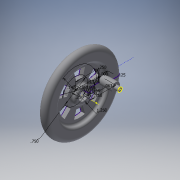
# Autodesk Inventor part: Caufield_Wheel
Saved by Autodesk Inventor 2016 (Build 200138000, 138)
## iProperties
Created: 2018-01-11
Part Number: Caufield_Wheel
Material: Generic
Document SubType Name: Modeling
Designer: The Panda
Density: 1 g/cm^3
Appearance: Default
Mass: 11.5444 g
Surface Area: 63.3015 cm^2
Volume: 11.5444 cm^3
Author: The Panda
Autodesk Inventor part; units mm, degrees
ref_plane "XZ Plane" through (0, 0, 0) normal (0, 1, 0) x (-1, 0, 0)
ref_plane "XY Plane" through (0, 0, 0) normal (0, 0, 1) x (1, 0, 0)
sketch "Wheel sketch" plane through (0, 0, 0) normal (0, 0, 1) x (1, 0, 0)
  line L0 (0, 0) -> (0, 6.4629) construction
  line L1 (3.556, 0) -> (3.556, 6.35)
  line L2 (25.4, 6.35) -> (25.4, 0) construction
  line L3 (25.4, 0) -> (3.556, 0)
  arc A0 (25.4, 0) -> (25.4, 6.35) centre (25.4, 3.175) ccw
  line L4 (0, 0) -> (43.9358, 0) construction
  line L5 (3.556, 6.35) -> (4.7625, 6.35)
  line L6 (6.35, 4.7625) -> (6.35, 4.7625)
  line L7 (7.9375, 3.175) -> (17.4625, 3.175)
  line L8 (25.4, 6.35) -> (20.6375, 6.35)
  line L9 (19.05, 4.7625) -> (19.05, 4.7625)
  arc A1 (6.35, 4.7625) -> (4.7625, 6.35) centre (4.7625, 4.7625) ccw
  arc A2 (6.35, 4.7625) -> (7.9375, 3.175) centre (7.9375, 4.7625) ccw
  arc A3 (17.4625, 3.175) -> (19.05, 4.7625) centre (17.4625, 4.7625) ccw
  arc A4 (20.6375, 6.35) -> (19.05, 4.7625) centre (20.6375, 4.7625) ccw
  point P0 (6.35, 6.35)
  point P1 (6.35, 3.175)
  point P2 (19.05, 3.175)
  point P3 (19.05, 6.35)
  dimension "d3" = 3.175
  dimension "d4" = 25.4
  dimension "d5" = 3.556
  dimension "d6" = 6.35
  dimension "d7" = 6.35
  dimension "d8" = 3.175
  dimension "d9" = 19.05
  dimension "d11" = 1.5875
  constraints: 20 end point, 10 point on circle, 9 point on line, 8 tangent, 5 centre point, 4 horizontal, 3 equal radius, 3 vertical, 2 perpendicular, 1 collinear, 1 midpoint
  measures "d3" radius of A0
  measures "d4" horizontal distance of A0.centre L0.start
  measures "d5" distance between parallel lines of L0 L1
  measures "d6" distance from line of point (6.35, 6.35) L0
  measures "d7" distance of L1.start L1.end
  measures "d8" distance of point (6.35, 6.35) point (6.35, 3.175)
  measures "d9" distance from line of L0 point (19.05, 3.175)
  measures "d11" radius of A1
revolve "Wheel revolution" add sketch "Wheel sketch" angle 360 about axis through (0, 0, 0) along (0, 1, 0)
sketch "spoke and peg sketch" plane through (0, 0, 0) normal (0, -1, 0) x (1, 0, 0)
  circle A0 centre (0, 0) radius 3.556 projected
  circle A1 centre (0, 0) radius 25.4 projected
  line L0 (0, 0) -> (17.78, 0) construction
  arc A2 (9.2004, 2.4653) -> (6.7352, 6.7352) centre (0, 0) ccw
  circle A3 centre (0, 0) radius 4.7625 construction
  arc A4 (15.3341, 4.1088) -> (11.2253, 11.2253) centre (0, 0) ccw
  line L1 (6.7352, 6.7352) -> (11.2253, 11.2253)
  line L2 (9.2004, 2.4653) -> (15.3341, 4.1088)
  line L3 (6.7352, 6.7352) -> (0, 0) construction
  line L4 (0, 0) -> (9.2004, 2.4653) construction
  line L5 (2.4653, 9.2004) -> (4.1088, 15.3341)
  arc A5 (4.1088, 15.3341) -> (-4.1088, 15.3341) centre (0, 0) ccw
  line L6 (-2.4653, 9.2004) -> (-4.1088, 15.3341)
  arc A6 (2.4653, 9.2004) -> (-2.4653, 9.2004) centre (0, 0) ccw
  line L7 (-6.7352, 6.7352) -> (-11.2253, 11.2253)
  arc A7 (-11.2253, 11.2253) -> (-15.3341, 4.1088) centre (0, 0) ccw
  line L8 (-9.2004, 2.4653) -> (-15.3341, 4.1088)
  arc A8 (-6.7352, 6.7352) -> (-9.2004, 2.4653) centre (0, 0) ccw
  line L9 (-9.2004, -2.4653) -> (-15.3341, -4.1088)
  arc A9 (-15.3341, -4.1088) -> (-11.2253, -11.2253) centre (0, 0) ccw
  line L10 (-6.7352, -6.7352) -> (-11.2253, -11.2253)
  arc A10 (-9.2004, -2.4653) -> (-6.7352, -6.7352) centre (0, 0) ccw
  line L11 (-2.4653, -9.2004) -> (-4.1088, -15.3341)
  arc A11 (-4.1088, -15.3341) -> (4.1088, -15.3341) centre (0, 0) ccw
  line L12 (2.4653, -9.2004) -> (4.1088, -15.3341)
  arc A12 (-2.4653, -9.2004) -> (2.4653, -9.2004) centre (0, 0) ccw
  line L13 (6.7352, -6.7352) -> (11.2253, -11.2253)
  arc A13 (11.2253, -11.2253) -> (15.3341, -4.1088) centre (0, 0) ccw
  line L14 (9.2004, -2.4653) -> (15.3341, -4.1088)
  arc A14 (6.7352, -6.7352) -> (9.2004, -2.4653) centre (0, 0) ccw
  circle A15 centre (17.78, 0) radius 3.175
  circle A16 centre (17.78, 0) radius 1.5875
  dimension "d14" = 19.05
  dimension "d15" = 31.75
  dimension "d16" = 15
  dimension "d17" = 30
  dimension "d18" = 30
  dimension "d21" = 360
  dimension "d25" = 17.78
  dimension "d26" = 6.35
  dimension "d27" = 3.175
  constraints: 30 end point, 24 point on circle, 14 centre point, 5 coincident, 1 collinear, 1 horizontal, 61 other
  measures "d14" diameter of A2
  measures "d15" diameter of A4
  measures "d16" angle of L0 L2
  measures "d17" angle of L1 L2
  measures "d18" angle of L4 L3
  measures "d25" distance of L0.start L0.end
  measures "d26" diameter of A15
  measures "d27" diameter of A16
extrude "Wheel spoke Extrusion" cut sketch "spoke and peg sketch" against normal blind 6.35 contours A2 L1 A4 L2 | A6 L6 A5 L5 | A8 L8 A7 L7 | A10 L10 A9 L9 | A12 L12 A11 L11 | A14 L14 A13 L13
extrude "Thick peg extrution" add sketch "spoke and peg sketch" against normal blind 12.7 contours A15
extrude "thin peg extrution" add sketch "spoke and peg sketch" against normal blind 15.875 contours A16
sketch "Peg hole point sketch" plane through (17.78, 15.875, 0) normal (0, 1, 0) x (1, 0, 0)
  circle A0 centre (0, 0) radius 1.5875 projected
  point P0 (-17.78, 0)
  constraints: 1 coincident
hole "Peg hole" at (17.78, 15.875, 0) direction (0, -1, 0) diameter 1.5875 depth 6.35
body "Solid1"
